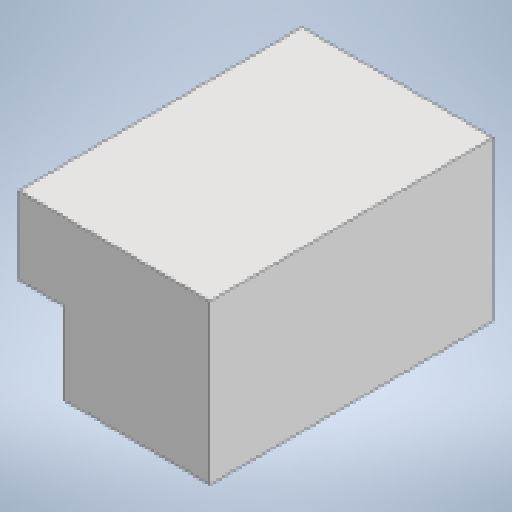
# Autodesk Inventor part: uchwyt_serwa_czlon0_pre
Saved by Autodesk Inventor 2023 (Build 270158000, 158)
## iProperties
Created: 2024-06-29
Part Number: uchwyt_serwa_czlon0_pre
Material: Ogólny
Document SubType Name: Modeling
Designer: kamil
Density: 1 g/cm^3
Appearance: Domyślna
Author: kamil
Autodesk Inventor part; units mm, degrees
ref_plane "YZ Plane" through (0, 0, 0) normal (1, 0, 0) x (0, 1, 0)
ref_plane "XZ Plane" through (0, 0, 0) normal (0, 1, 0) x (-1, 0, 0)
ref_plane "XY Plane" through (0, 0, 0) normal (0, 0, 1) x (1, 0, 0)
sketch "Szkic1" plane through (0, 0, 0) normal (0, 1, 0) x (-1, 0, 0)
  line L0 (21.577, 10.8523) -> (-8.423, 10.8523)
  line L1 (-8.423, 10.8523) -> (-8.423, -31.1477)
  line L2 (-8.423, -31.1477) -> (21.577, -31.1477)
  line L3 (21.577, 18.8523) -> (-16.423, 18.8523)
  line L4 (-16.423, 18.8523) -> (-16.423, -39.1477)
  line L5 (-16.423, -39.1477) -> (21.577, -39.1477)
  line L6 (21.577, 10.8523) -> (21.577, 18.8523)
  line L7 (21.577, -31.1477) -> (21.577, -39.1477)
  point P0 (0, 0)
  dimension "d0" = 42
  dimension "d1" = 30
  dimension "d2" = 8
  constraints: 16 end point, 3 equal length, 2 perpendicular, 1 horizontal, 1 vertical, 2 other
  measures "d0" distance of L1.end L0.end
  measures "d1" distance of L0.start L0.end
  measures "d2" distance between parallel lines of L0 L3
extrude "Wyciągnięcie proste1" add sketch "Szkic1" along normal blind 22
sketch "Szkic2" plane through (0, 22, 0) normal (0, 1, 0) x (1, 0, 0)
  line L0 (16.423, 39.1477) -> (-21.577, 39.1477) projected
  line L1 (16.423, 39.1477) -> (-32.877, 39.1477)
  line L2 (-32.877, 39.1477) -> (-32.877, -18.8523)
  line L3 (-32.877, -18.8523) -> (16.423, -18.8523)
  line L4 (16.423, -18.8523) -> (16.423, 39.1477)
  point P0 (0, 0)
  dimension "d5" = 49.3
  constraints: 8 end point, 2 parallel, 1 horizontal, 1 perpendicular
  measures "d5" distance between parallel lines of L2 L4
extrude "Wyciągnięcie proste2" add sketch "Szkic2" along normal blind 15
sketch "Szkic3" plane through (16.423, 0, 18.8523) normal (1, 0, 0) x (0, 0, -1)
  line L0 (0, 0) -> (58, 0) projected
  line L1 (58, 0) -> (58, 37) projected
  line L2 (0, 37) -> (58, 37) projected
  line L3 (0, 0) -> (0, 37) projected
  line L4 (0, 37) -> (-15, 37)
  line L5 (-15, 37) -> (-15, 0)
  line L6 (-15, 0) -> (0, 0)
  line L7 (0, 0) -> (0, 37)
  line L8 (58, 37) -> (73, 37)
  line L9 (73, 37) -> (73, 0)
  line L10 (73, 0) -> (58, 0)
  line L11 (58, 0) -> (58, 37)
  point P0 (18.8523, 0)
  dimension "d8" = 15
  dimension "d9" = 15
  constraints: 16 end point, 4 parallel, 2 horizontal, 2 perpendicular, 1 horizontal alignment, 1 point on line
  measures "d8" distance of L6.end L5.end
  measures "d9" distance of L9.end L10.end
extrude "Wyciągnięcie proste3" add sketch "Szkic3" against normal up to surface (49.3 mm away) contours L6 L5 L4 L3 | L1 L8 L9 L10
sketch "Szkic4" plane through (0, 0, 0) normal (0, -1, 0) x (1, 0, 0)
  line L0 (16.423, 33.8523) -> (16.423, -54.1477) projected
  line L1 (16.423, 33.8523) -> (-32.877, 33.8523) projected
  line L2 (-32.877, 33.8523) -> (-32.877, 18.8523) projected
  line L3 (-21.577, 18.8523) -> (-32.877, 18.8523) projected
  line L4 (-21.577, 10.8523) -> (-21.577, 18.8523) projected
  line L5 (8.423, 10.8523) -> (-21.577, 10.8523) projected
  line L6 (8.423, -31.1477) -> (8.423, 10.8523) projected
  line L7 (-21.577, -31.1477) -> (8.423, -31.1477) projected
  line L8 (-21.577, -39.1477) -> (-21.577, -31.1477) projected
  line L9 (-21.577, -39.1477) -> (-32.877, -39.1477) projected
  line L10 (-32.877, -39.1477) -> (-32.877, -54.1477) projected
  line L11 (16.423, -54.1477) -> (-32.877, -54.1477) projected
  point P0 (0, 0)
extrude "Wyciągnięcie proste4" cut sketch "Szkic4" against normal blind 1
sketch "Szkic5" plane through (-32.877, 22, -39.1477) normal (-1, 0, 0) x (0, 0, 1)
  line L0 (-15, -21) -> (0, -21) projected
  line L1 (0, 0) -> (0, -21) projected
  line L2 (0, 0) -> (58, 0) projected
  line L3 (58, -21) -> (58, 0) projected
  line L4 (58, -21) -> (73, -21) projected
  line L5 (73, 15) -> (73, -21) projected
  line L6 (-15, 15) -> (73, 15) projected
  line L7 (-15, -21) -> (-15, 15) projected
  line L8 (0, 0) -> (0, 15)
  point P0 (39.1477, -22)
  constraints: 2 end point, 1 point on line, 1 vertical
extrude "Wyciągnięcie proste5" cut sketch "Szkic5" against normal through all contours L7 L6 L8 L1 L0
